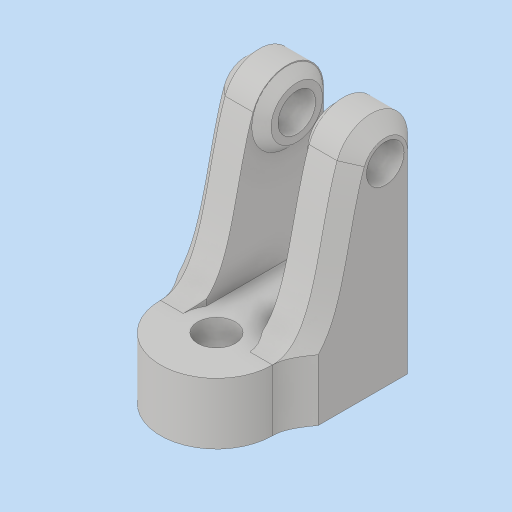
# Autodesk Inventor part: Profil-WheelHoldVert-wBearing
Saved by Autodesk Inventor 2024 (Build 280153000, 153)
## iProperties
Created: 2023-04-19
Part Number: Profil-WheelHoldVert-wBearing
Material: Generic
Document SubType Name: Modeling
Designer: Karbosch
Density: 1 g/cm^3
Appearance: Default
Mass: 3.67486 g
Surface Area: 22.487 cm^2
Volume: 3.67486 cm^3
Author: Karbosch
Autodesk Inventor part; units mm, degrees
note: some values were not read from the file. Chosen so that the rebuilt part matches the saved one: edges of "Chamfer6".
ref_plane "XZ Plane" through (0, 0, 0) normal (0, 1, 0) x (-1, 0, 0)
ref_plane "XY Plane" through (0, 0, 0) normal (0, 0, 1) x (1, 0, 0)
ref_plane "Work Plane1" through (8, 0, 0) normal (1, 0, 0) x (0, 1, 0)
sketch "Sketch2" plane through (8, -3.3137, 0) normal (1, 0, 0) x (0, 0, -1)
  circle A0 centre (0, 25.4137) radius 2.15
  circle A1 centre (0, 25.4137) radius 4.15
  circle A2 centre (0, 25.4137) radius 11
  circle A3 centre (0, 25.4137) radius 8.1
  line L0 (-15.8398, 3.3137) -> (15.4733, 3.3137) projected
  line L1 (-3.8997, 26.8331) -> (-6.2789, 20.2965) construction
  line L2 (-6.2789, 20.2965) -> (-6.2789, 10.3137) construction
  line L3 (-6.2789, 10.3137) -> (-11.2789, 10.3137) construction
  spline S0 degree 3 poles (-3.8997, 26.8331) (-6.2789, 20.2965) (-6.2789, 10.3137) (-11.2789, 10.3137) knots 1 1 1 1 2 2 2 2
  line L4 (4.15, 25.4137) -> (4.15, 10.3137)
  line L5 (4.15, 10.3137) -> (-11.2789, 10.3137)
  point P0 (0, 3.3137)
  dimension "d33" = 16.2
  dimension "d4" = 4.3
  dimension "d6" = 2
  dimension "d19" = 22
  dimension "d37" = 14
  dimension "d38" = 7
  dimension "d40" = 160
  dimension "d48" = 5
  constraints: 4 end point, 3 centre point, 3 coincident, 2 point on circle, 2 tangent, 2 vertical, 1 horizontal alignment, 1 perpendicular, 1 vertical alignment, 6 other
  measures "d4" diameter of A0
  measures "d6" radial gap between concentric circles of A1 A0
  measures "d19" diameter of A2
  measures "d38" distance from line of L0 L3.end
  measures "d40" angle of L1 L2
  measures "d48" distance of L2.end L3.end
extrude "Extrusion2" add sketch "Sketch2" against normal blind 4.8 contours A1 | L4 A3 S0 A1 | L4 A2 S0 A3 | L4 L5 S0 A2 picked at (1.5398, 18.8491) picked at (-5.1375, 16.8414)
sketch "Sketch5" plane through (3.2, -3.3137, 0) normal (-1, 0, 0) x (0, 0, 1)
  circle A0 centre (0, 25.4137) radius 2.15 projected
  circle A1 centre (0, 25.4137) radius 2.95
  point P0 (0, 3.3137)
  dimension "d41" = 0.8
  constraints: 1 centre point, 1 coincident
  measures "d41" radial gap between concentric circles of A1 A0
extrude "Extrusion5" add sketch "Sketch5" along normal blind 1.1
chamfer "Chamfer5" distance 1.1 angle 45 1 edges at (3.2, 22.1, -2.95)
chamfer "Chamfer6" distance 1.6 angle 45 2 edges at (8, 26.187, -0.7206) (8, 12.8085, 6.6065)
mirror "Mirror3" about plane through (0, 0, 0) normal (1, 0, 0) of "Extrusion2", "Extrusion5", "Chamfer5", "Chamfer6"
sketch "Sketch6" plane through (0, 0, 0) normal (0, 1, 0) x (-1, 0, 0)
  line L0 (6.4, -4.15) -> (8, -2.55) projected
  line L1 (6.4, -4.15) -> (3.2, -4.15) projected
  line L2 (3.2, -4.15) -> (3.2, 11.2789) projected
  line L3 (6.4, 11.2789) -> (3.2, 11.2789) projected
  spline S0 degree 8 poles (8, 7.6489) (7.9505, 7.717) (7.9011, 7.7857) (7.8517, 7.855) (7.8023, 7.9249) (7.7529, 7.9955) (7.7035, 8.0668) (7.6541, 8.1389) (7.5557, 8.2846) (7.5066, 8.3582) (7.4575, 8.4328) (7.4085, 8.5085) (7.3595, 8.5853) (7.3106, 8.6634) (7.2617, 8.7431) (7.1592, 8.9138) (7.1057, 9.0052) (7.0523, 9.099) (6.9989, 9.1955) (6.9457, 9.2954) (6.8926, 9.3993) (6.8398, 9.5081) (6.7593, 9.6851) (6.7315, 9.7484) (6.7038, 9.8139) (6.6762, 9.882) (6.6488, 9.953) (6.6216, 10.0278) (6.5946, 10.1069) (6.554, 10.2373) (6.5401, 10.284) (6.5263, 10.3327) (6.5127, 10.3837) (6.4992, 10.4372) (6.4861, 10.494) (6.4732, 10.5545) (6.4541, 10.6561) (6.4475, 10.6937) (6.441, 10.733) (6.4348, 10.7742) (6.4288, 10.8177) (6.4233, 10.8635) (6.4181, 10.9122) (6.4119, 10.983) (6.4104, 11.0022) (6.4089, 11.0214) (6.4076, 11.0406) (6.4064, 11.0599) (6.4053, 11.0791) (6.4044, 11.0984) (6.4027, 11.1371) (6.4019, 11.1568) (6.4013, 11.1768) (6.4008, 11.197) (6.4004, 11.2174) (6.4001, 11.2378) (6.4, 11.2582) (6.4, 11.2789) knots 0 0 0 0 0 0 0 0 0 0.234274 0.234274 0.234274 0.234274 0.234274 0.234274 0.234274 0.467508 0.467508 0.467508 0.467508 0.467508 0.467508 0.467508 0.723386 0.723386 0.723386 0.723386 0.723386 0.723386 0.723386 0.859248 0.859248 0.859248 0.859248 0.859248 0.859248 0.859248 0.931051 0.931051 0.931051 0.931051 0.931051 0.931051 0.931051 0.970673 0.970673 0.970673 0.970673 0.970673 0.970673 0.970673 0.985351 0.985351 0.985351 0.985351 0.985351 0.985351 0.985351 1 1 1 1 1 1 1 1 1 projected
  line L4 (8, 7.6489) -> (8, -2.55) projected
  line L5 (-8, -2.55) -> (-6.4, -4.15) projected
  line L6 (-8, 7.6489) -> (-8, -2.55) projected
  spline S1 degree 8 poles (-6.4, 11.2789) (-6.4, 11.2582) (-6.4001, 11.2378) (-6.4004, 11.2174) (-6.4008, 11.197) (-6.4013, 11.1768) (-6.4019, 11.1568) (-6.4027, 11.1371) (-6.4044, 11.0984) (-6.4053, 11.0791) (-6.4064, 11.0599) (-6.4076, 11.0406) (-6.4089, 11.0214) (-6.4104, 11.0022) (-6.4119, 10.983) (-6.4181, 10.9122) (-6.4233, 10.8635) (-6.4288, 10.8177) (-6.4348, 10.7742) (-6.441, 10.733) (-6.4475, 10.6937) (-6.4541, 10.6561) (-6.4732, 10.5545) (-6.4861, 10.494) (-6.4992, 10.4372) (-6.5127, 10.3837) (-6.5263, 10.3327) (-6.5401, 10.284) (-6.554, 10.2373) (-6.5946, 10.1069) (-6.6216, 10.0278) (-6.6488, 9.953) (-6.6762, 9.882) (-6.7038, 9.8139) (-6.7315, 9.7484) (-6.7593, 9.6851) (-6.8398, 9.5081) (-6.8926, 9.3993) (-6.9457, 9.2954) (-6.9989, 9.1955) (-7.0523, 9.099) (-7.1057, 9.0052) (-7.1592, 8.9138) (-7.2617, 8.7431) (-7.3106, 8.6634) (-7.3595, 8.5853) (-7.4085, 8.5085) (-7.4575, 8.4328) (-7.5066, 8.3582) (-7.5557, 8.2846) (-7.6541, 8.1389) (-7.7035, 8.0668) (-7.7529, 7.9955) (-7.8023, 7.9249) (-7.8517, 7.855) (-7.9011, 7.7857) (-7.9505, 7.717) (-8, 7.6489) knots 0 0 0 0 0 0 0 0 0 0.014649 0.014649 0.014649 0.014649 0.014649 0.014649 0.014649 0.029327 0.029327 0.029327 0.029327 0.029327 0.029327 0.029327 0.068949 0.068949 0.068949 0.068949 0.068949 0.068949 0.068949 0.140752 0.140752 0.140752 0.140752 0.140752 0.140752 0.140752 0.276614 0.276614 0.276614 0.276614 0.276614 0.276614 0.276614 0.532492 0.532492 0.532492 0.532492 0.532492 0.532492 0.532492 0.765726 0.765726 0.765726 0.765726 0.765726 0.765726 0.765726 1 1 1 1 1 1 1 1 1 projected
  line L7 (-6.4, 11.2789) -> (-3.2, 11.2789) projected
  line L8 (-3.2, -4.15) -> (-3.2, 11.2789) projected
  line L9 (-6.4, -4.15) -> (-3.2, -4.15) projected
  line L10 (6.4, 11.2789) -> (3.2, 11.2789) projected
  arc A0 (6.4, 11.2789) -> (-6.4, 11.2789) centre (0, 11.2789) ccw
  circle A1 centre (0, 11.2789) radius 2.15
  line L11 (-3.2, -4.15) -> (3.2, -4.15)
  point P0 (0, 0)
  dimension "d49" = 4.3
  constraints: 2 centre point, 2 end point, 2 point on circle, 1 coincident, 1 horizontal, 1 horizontal alignment, 2 other
  measures "d49" diameter of A1
extrude "Extrusion6" add sketch "Sketch6" along normal up to surface (7 mm away)
sketch "Sketch7" plane through (0, 7, 11.2789) normal (0, 1, 0) x (1, 0, 0)
  circle A0 centre (0, 0) radius 2.15 projected
  circle A1 centre (0, 0) radius 3.8
  point P0 (0, 11.2789)
  dimension "d52" = 7.6
  constraints: 1 centre point, 1 coincident
  measures "d52" diameter of A1
extrude "Extrusion7" cut sketch "Sketch7" along normal through all
sketch "Sketch8" plane through (0, 0, 0) normal (0, -1, 0) x (1, 0, 0)
  circle A0 centre (0, 11.2789) radius 2.15 projected
  line L0 (6.4, -4.15) -> (-6.4, -4.15) projected
  line L1 (2.5, -4.15) -> (-2.5, -4.15)
  line L2 (-2.5, -4.15) -> (-2.5, 4.7289)
  line L3 (-2.5, 4.7289) -> (2.5, 4.7289)
  line L4 (2.5, 4.7289) -> (2.5, -4.15)
  point P0 (0, 0)
  point P1 (0, -4.15)
  dimension "d55" = 5
  dimension "d56" = 4.4
  constraints: 8 end point, 2 midpoint, 2 parallel, 1 horizontal, 1 perpendicular, 1 point on line
  measures "d55" distance of L2.end L3.end
  measures "d56" distance edge to line of A0 L3
extrude "Extrusion8" add sketch "Sketch8" along normal blind 1.6 contours L0 L2 L3 L4
fillet "Fillet1" radius 0.4 3 edges at (2.5, 0, 0.2894) (-2.5, 0, 0.2894) (0, -1.6, 4.7289)
body "Solid1"
